Autodesk Inventor part; units mm, degrees
(part 2 of 2)
sketch "Sketch5" plane through (27.4, 0, -9.3) normal (0, 0, -1) x (-1, 0, 0)
  line L0 (24.9, -17.5) -> (27.4, -17.5) projected
  line L1 (24.9, -1) -> (24.9, -17.5) projected
  line L2 (27.4, -1) -> (24.9, -1) projected
  line L3 (27.4, -17.5) -> (27.4, -65.8371) projected
  line L4 (0, 0) -> (27.4, 0) projected
  line L5 (0, -6.5) -> (0, 0) projected
  line L6 (4.3, -6.5) -> (0, -6.5) projected
  line L7 (4.3, -65.8371) -> (4.3, -6.5) projected
  line L8 (27.4, -65.8371) -> (9.3323, -65.8371) projected
  line L9 (27.4, 0) -> (27.4, -1) projected
  arc A0 (10.6233, -44.2391) -> (10.8043, -51.0104) centre (18.398, -47.4193) ccw projected
  arc A1 (23.4456, -40.7049) -> (10.6233, -44.2391) centre (15.05, -35.2722) ccw projected
  arc A2 (17.6977, -55.79) -> (23.4456, -40.7049) centre (18.398, -47.4193) ccw projected
  arc A3 (10.8043, -51.0104) -> (17.6977, -55.79) centre (12.7, -55.6371) ccw projected
  circle A4 centre (7.0431, -49.9802) radius 2.25 projected
  circle A5 centre (18.3569, -61.2939) radius 2.25 projected
  circle A6 centre (7.55, -9.75) radius 3.25
  line L10 (24.9, -6.5) -> (4.3, -6.5)
  line L11 (24.9, -1) -> (24.9, -17.5) projected
  circle A7 centre (17.55, -9.75) radius 3.25
  line L12 (4.3, -65.8371) -> (4.3, -6.5) projected
  circle A8 centre (23.4, -24.0349) radius 4
  line L13 (27.4, -17.5) -> (27.4, -65.8371) projected
  circle A9 centre (23.9, -57.971) radius 3.5
  circle A10 centre (7.527, -45.2549) radius 2.5
  arc A11 (23.4456, -40.7049) -> (10.6233, -44.2391) centre (15.05, -35.2722) ccw projected
  line L14 (4.3, -19.5) -> (24.9, -19.5)
  circle A12 centre (9.4248, -23) radius 3.5
  circle A13 centre (7.527, -45.2549) radius 2.5
  line L15 (9.3323, -65.3371) -> (9.3323, -65.8371) projected
  line L16 (6.0157, -65.8371) -> (4.3, -65.8371) projected
  line L17 (6.0157, -65.8371) -> (6.0157, -65.3371) projected
  line L18 (6.0157, -65.3371) -> (9.3323, -65.3371) projected
  point P0 (27.4, 0)
  point P1 (27.4, -15)
  dimension "d124" = 6.5
  dimension "d125" = 6.5
  dimension "d126" = 6.5
  dimension "d127" = 10
  dimension "d128" = 8
  dimension "d129" = 7
  dimension "d130" = 5
  dimension "d133" = 19.5
  dimension "d141" = 7
  dimension "d178" = 5
  constraints: 11 tangent, 7 centre point, 4 end point, 4 point on line, 2 perpendicular, 1 coincident
  measures "d124" diameter of A6
  measures "d125" distance between parallel lines of L4 L10
  measures "d126" diameter of A7
  measures "d127" distance of A6.centre A7.centre
  measures "d128" diameter of A8
  measures "d129" diameter of A9
  measures "d130" diameter of A10
  measures "d133" distance between parallel lines of L14 L4
  measures "d141" diameter of A12
  measures "d178" diameter of A13
hole "Hole3" at (3.5, -57.971, -9.3) at (4, -24.0349, -9.3) at (19.873, -45.2549, -9.3) at (19.85, -9.75, -9.3) at (9.85, -9.75, -9.3) at (17.9752, -23, -9.3) direction (0, 0, 1) diameter 4 depth 4 counterbore diameter 6 counterbore depth 0.5
sketch "Sketch6" plane through (0, -65.8371, 0) normal (-1, 0, 0) x (0, 0, 1)
  circle A0 centre (2, 30.6685) radius 1.75 projected
  line L0 (0, 42.7371) -> (4, 42.7371) projected
  line L1 (0, 42.7371) -> (0, 18.6) projected
  line L2 (0, 18.6) -> (4, 18.6) projected
  line L3 (4, 42.7371) -> (4, 18.6) projected
  line L4 (2, 18.6) -> (2, 42.7371)
  line L5 (0, 30.6685) -> (4, 30.6685)
  point P0 (0, 65.8371)
  point P1 (2, 30.6685)
  constraints: 5 midpoint, 4 end point
hole "Hole4" at (0, -35.1685, 2) direction (1, 0, 0) diameter 2.9 end through all countersink diameter 6 countersink angle 90 clearance for "Countersunk Flat Head Screw ISO 2009/7046" size "M2.5" standard "ISO"
sketch "Sketch8" plane through (27.4, -6.5, -9.3) normal (1, 0, 0) x (0, 0, -1)
  line L0 (-5.3, 3.9525) -> (-5.3, 0) projected
  line L1 (-5.3, 0) -> (0, 0) projected
  line L2 (0, 0) -> (0, 6.5) projected
  line L3 (-9.3, 6.5) -> (0, 6.5) projected
  line L4 (-9.3, 3.9525) -> (-9.3, 6.5) projected
  line L5 (-9.3, 3.9525) -> (-5.3, 3.9525) projected
  line L6 (-5.3, 0) -> (0, 6.5)
  point P0 (-9.3, 6.5)
  point P1 (-2.65, 3.25)
  constraints: 2 end point, 1 midpoint
hole "Hole6" at (27.4, -3.25, -6.65) direction (-1, 0, 0) diameter 4 depth 6.5 counterbore diameter 4.5 counterbore depth 0.5
sketch "Sketch9" plane through (23.1, -65.8371, -9.3) normal (1, 0, 0) x (0, 0, -1)
  line L0 (-5.3, 58.882) -> (-9.3, 58.882) projected
  line L1 (-9.3, 47.6348) -> (-9.3, 58.882) projected
  line L2 (-9.3, 47.6348) -> (-5.3, 47.6348) projected
  line L3 (-9.3, 58.882) -> (0, 58.882)
  line L4 (0, 58.882) -> (0, 47.6348)
  line L5 (0, 47.6348) -> (-9.3, 47.6348)
  line L6 (-9.3, 47.6348) -> (-9.3, 58.882)
  line L7 (-5.3, 39.318) -> (-9.3, 39.318) projected
  line L8 (-9.3, 0) -> (-9.3, 39.318) projected
  line L9 (-9.3, 0) -> (0, 0) projected
  line L10 (0, 0) -> (0, 59.3371) projected
  line L11 (-5.3, 59.3371) -> (0, 59.3371) projected
  line L12 (-5.3, 59.3371) -> (-5.3, 58.882) projected
  line L13 (-5.3, 58.882) -> (-9.3, 58.882) projected
  line L14 (-9.3, 47.6348) -> (-9.3, 58.882) projected
  line L15 (-9.3, 47.6348) -> (-5.3, 47.6348) projected
  line L16 (-5.3, 47.6348) -> (-5.3, 39.318) projected
  circle A0 centre (-3.3, 52.2136) radius 2.75
  circle A1 centre (-6.55, 2.75) radius 2.75
  circle A2 centre (-3.3, 52.2136) radius 2
  line L17 (-4, 54.0871) -> (-4, 58.0871) projected
  line L18 (-5.3, 46.1371) -> (-5.3, 56.1371) projected
  point P0 (-9.3, 65.8371)
  dimension "d174" = 4
  dimension "d165" = 5.5
  dimension "d173" = 5.5
  constraints: 8 end point, 2 centre point, 2 parallel, 2 point on line, 2 tangent, 1 coincident, 1 horizontal, 1 perpendicular, 1 vertical, 3 other
  measures "d165" diameter of A0
  measures "d173" diameter of A1
hole "Hole7" at (23.1, -13.6235, -6) at (23.1, -63.0871, -2.75) direction (-1, 0, 0) diameter 3 depth 5 counterbore diameter 3.5 counterbore depth 0.5
sketch "Sketch10" plane through (9.002, -47.4193, -1.6) normal (0, 0, -1) x (-1, 0, 0)
  circle A0 centre (0, 0) radius 4.6 projected
  circle A1 centre (0, 0) radius 1.25
  point P0 (9.002, 47.4193)
  dimension "d175" = 2.5
  constraints: 1 centre point, 1 coincident
  measures "d175" diameter of A1
extrude "Extrusion11" cut sketch "Sketch10" against normal blind 1.4 contours A1
fillet "Fillet1" radius 2 7 edges at (11.1977, -6.9551, -2) (6.7901, -2.5475, -2) (2.5475, -6.7901, -2) (6.9551, -11.1977, -2) (18.2023, -22.4449, -2) (22.6099, -26.8525, -2) (22.4449, -18.2023, -2)
sketch "Sketch11" plane through (27.4, 0, -9.3) normal (0, 0, -1) x (-1, 0, 0)
  line L0 (24.4, -45.7371) -> (24.4, -28.981) construction
  arc A0 (24.4, -45.7371) -> (25.9, -47.2371) centre (25.9, -45.7371) ccw construction
  line L1 (27.4, -47.2371) -> (25.9, -47.2371) construction
  line L2 (27.4, -37.056) -> (27.4, -39.867) construction
  line L3 (27.4, -40.6854) -> (27.4, -47.2371) construction
  circle A1 centre (25.9569, -40.2762) radius 2
  circle A2 centre (25.9, -28.981) radius 2.542 construction
  circle A3 centre (18.3569, -61.2939) radius 2.25
  arc A4 (8.3411, -48.1424) -> (10.012, -46.9357) centre (7.527, -45.2549) ccw
  arc A5 (6.1446, -47.9174) -> (8.3411, -48.1424) centre (7.0431, -49.9802) ccw
  arc A6 (7.9165, -42.2803) -> (6.1446, -47.9174) centre (7.527, -45.2549) ccw
  arc A7 (23.4456, -40.7049) -> (7.9165, -42.2803) centre (15.05, -35.2722) ccw
  arc A8 (17.6977, -55.79) -> (23.4456, -40.7049) centre (18.398, -47.4193) ccw
  arc A9 (10.8043, -51.0104) -> (17.6977, -55.79) centre (12.7, -55.6371) ccw
  arc A10 (10.012, -46.9357) -> (10.8043, -51.0104) centre (18.398, -47.4193) ccw
  line L4 (9.3323, -65.3371) -> (9.3323, -65.8371)
  line L5 (27.4, -65.8371) -> (9.3323, -65.8371)
  line L6 (27.4, -17.5) -> (27.4, -65.8371)
  line L7 (24.9, -17.5) -> (27.4, -17.5)
  line L8 (24.9, -1) -> (24.9, -17.5)
  line L9 (27.4, -1) -> (24.9, -1)
  line L10 (27.4, 0) -> (27.4, -1)
  line L11 (0, 0) -> (27.4, 0)
  line L12 (0, -6.5) -> (0, 0)
  line L13 (4.3, -6.5) -> (0, -6.5)
  line L14 (4.3, -65.8371) -> (4.3, -6.5)
  line L15 (6.0157, -65.8371) -> (4.3, -65.8371)
  line L16 (6.0157, -65.8371) -> (6.0157, -65.3371)
  line L17 (6.0157, -65.3371) -> (9.3323, -65.3371)
  circle A11 centre (23.9, -57.971) radius 3
  circle A12 centre (23.4, -24.0349) radius 3
  circle A13 centre (7.55, -9.75) radius 3
  circle A14 centre (17.55, -9.75) radius 3
  circle A15 centre (9.4248, -23) radius 3
  circle A16 centre (25.9569, -40.2762) radius 1
  circle A17 centre (25.9, -28.981) radius 1
  arc A18 (23.4456, -40.7049) -> (7.9165, -42.2803) centre (15.05, -35.2722) ccw
  circle A19 centre (23.4, -24.0349) radius 3
  circle A20 centre (25.9, -28.981) radius 2
  arc A21 (17.6977, -55.79) -> (23.4456, -40.7049) centre (18.398, -47.4193) ccw
  circle A22 centre (23.4, -24.0349) radius 2
  circle A23 centre (23.4, -24.0349) radius 3.25 construction
  arc A24 (24.4, -28.981) -> (27.4, -28.981) centre (25.9, -28.981) ccw
  arc A25 (27.4, -39.867) -> (27.4, -40.6854) centre (25.9569, -40.2762) ccw
  line L18 (27.4, -28.981) -> (27.4, -33.2811)
  spline S0 degree 2 poles (27.4, -37.056) (26.1045, -35.1685) (27.4, -33.2811) knots 0 0 0 1 1 1 weights 1 1.375 1
  point P0 (27.4, 0)
  dimension "d180" = 5.084
  dimension "d181" = 4
  dimension "d182" = 2
  dimension "d183" = 2
  dimension "d184" = 1.5569
  dimension "d185" = 1.4431
  dimension "d186" = 1.5
  dimension "d187" = 1.5
  dimension "d188" = 4
  dimension "d196" = 6.5
  constraints: 6 centre point, 4 coincident, 4 tangent
  measures "d180" diameter of A2
  measures "d181" diameter of A1
  measures "d182" diameter of A16
  measures "d183" diameter of A17
  measures "d184" distance from line of L0 A16.centre
  measures "d185" distance from line of L2 A1.centre
  measures "d186" distance from line of L0 A2.centre
  measures "d187" distance from line of L6 A2.centre
  measures "d188" diameter of A20
  measures "d196" diameter of A23
hole "Hole8" at (1.4431, -40.2762, -9.3) at (1.5, -28.981, -9.3) direction (0, 0, 1) diameter 2 end through all clearance for "Countersunk Flat Head Screw ISO 2009/7046" size "M2" standard "ISO"
body "Solid1"
